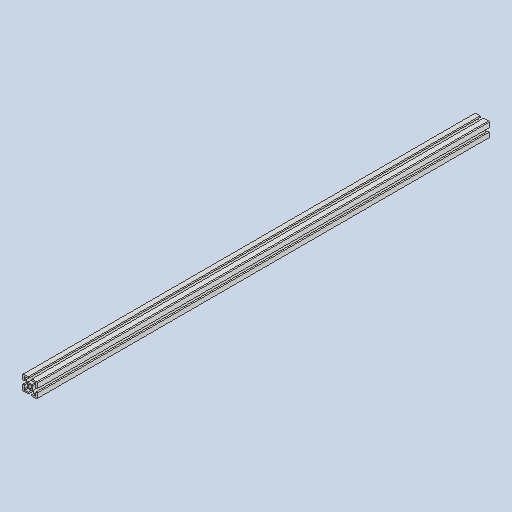
# Autodesk Inventor part: Perfil 20X20 T-622
Saved by Autodesk Inventor 2024.2 (Build 282272000, 272)
## iProperties
Created: 2024-08-23
Part Number: Perfil 20X20 T-622
Material: Generic
Document SubType Name: Modeling
Designer: ja.restrepo1
Density: 1 g/cm^3
Appearance: Default
Author: ja.restrepo1
Autodesk Inventor part; units mm, degrees
ref_plane "YZ Plane" through (0, 0, 0) normal (1, 0, 0) x (0, 1, 0)
ref_plane "XZ Plane" through (0, 0, 0) normal (0, 1, 0) x (-1, 0, 0)
ref_plane "XY Plane" through (0, 0, 0) normal (0, 0, 1) x (1, 0, 0)
sketch "Sketch1" plane through (0, 0, 0) normal (0, 0, 1) x (1, 0, 0)
  line L0 (9, 10) -> (2.5, 10)
  line L1 (-10, 9) -> (-10, 2.5)
  line L2 (-9, -10) -> (-2.5, -10)
  line L3 (10, -9) -> (10, -2.5)
  circle A0 centre (0, 0) radius 2.5
  line L4 (3.6, 3.6) -> (-3.6, 3.6) construction
  line L5 (-3.6, 3.6) -> (-3.6, -3.6) construction
  line L6 (-3.6, -3.6) -> (3.6, -3.6) construction
  line L7 (3.6, -3.6) -> (3.6, 3.6) construction
  line L8 (3.6, 3.6) -> (10, 10) construction
  line L9 (3.6, -3.6) -> (10, -10) construction
  line L10 (-3.6, -3.6) -> (-10, -10) construction
  line L11 (-10, 10) -> (-3.6, 3.6) construction
  line L12 (3.65, 2.8974) -> (8, 7.2474)
  line L13 (8, 7.2474) -> (8, 2.5)
  line L14 (8, 2.5) -> (10, 2.5)
  line L15 (10, 2.5) -> (10, -2.5) construction
  line L16 (10, -2.5) -> (8, -2.5)
  line L17 (8, -2.5) -> (8, -7.2474)
  line L18 (8, -7.2474) -> (3.65, -2.8974)
  line L19 (3.65, -2.8974) -> (3.65, 2.8974)
  line L20 (10, 2.5) -> (10, 9)
  line L21 (10, -2.5) -> (10, 2.5) construction
  line L22 (-2.5, 8) -> (-2.5, 10)
  line L23 (-7.2474, 8) -> (-2.5, 8)
  line L24 (-2.8974, 3.65) -> (-7.2474, 8)
  line L25 (2.8974, 3.65) -> (-2.8974, 3.65)
  line L26 (7.2474, 8) -> (2.8974, 3.65)
  line L27 (2.5, 8) -> (7.2474, 8)
  line L28 (2.5, 10) -> (2.5, 8)
  line L29 (-8, -2.5) -> (-10, -2.5)
  line L30 (-8, -7.2474) -> (-8, -2.5)
  line L31 (-3.65, -2.8974) -> (-8, -7.2474)
  line L32 (-3.65, 2.8974) -> (-3.65, -2.8974)
  line L33 (-8, 7.2474) -> (-3.65, 2.8974)
  line L34 (-8, 2.5) -> (-8, 7.2474)
  line L35 (-10, 2.5) -> (-8, 2.5)
  line L36 (2.5, -8) -> (2.5, -10)
  line L37 (7.2474, -8) -> (2.5, -8)
  line L38 (2.8974, -3.65) -> (7.2474, -8)
  line L39 (-2.8974, -3.65) -> (2.8974, -3.65)
  line L40 (-7.2474, -8) -> (-2.8974, -3.65)
  line L41 (-2.5, -8) -> (-7.2474, -8)
  line L42 (-2.5, -10) -> (-2.5, -8)
  line L43 (-2.5, -10) -> (2.5, -10) construction
  line L44 (2.5, -10) -> (9, -10)
  line L45 (-10, 2.5) -> (-10, -2.5) construction
  line L46 (-10, -2.5) -> (-10, -9)
  line L47 (-2.5, 10) -> (-9, 10)
  line L48 (2.5, 10) -> (-2.5, 10) construction
  arc A1 (-9, 10) -> (-10, 9) centre (-9, 9) ccw
  arc A2 (10, 9) -> (9, 10) centre (9, 9) ccw
  arc A3 (9, -10) -> (10, -9) centre (9, -9) ccw
  arc A4 (-10, -9) -> (-9, -10) centre (-9, -9) ccw
  point P0 (0, 0)
  point P1 (0, 3.6)
  point P2 (3.6, 0)
  point P3 (10, 0)
  point P4 (3.65, 0)
  point P5 (10, 0)
  point P6 (0, 3.65)
  point P7 (0, 3.65)
  point P8 (-3.65, 0)
  point P9 (0, -3.65)
  point P10 (0, 10)
  dimension "d2" = 5
  dimension "d3" = 7.2
  dimension "d4" = 7.2
  dimension "d5" = 2
  dimension "d6" = 6.35
  dimension "d7" = 4.7474
  dimension "d8" = 5
  dimension "d9" = 10
  dimension "d10" = 360
  dimension "d11" = 10
  dimension "d12" = 1
  constraints: 98 end point, 21 parallel, 16 perpendicular, 15 point on line, 8 point on circle, 8 tangent, 7 coincident, 7 midpoint, 5 centre point, 4 collinear, 4 horizontal, 4 horizontal alignment, 3 equal radius, 3 vertical alignment, 1 vertical, 65 other
  measures "d2" diameter of A0
  measures "d3" distance of L6.end L10.start
  measures "d4" distance of L10.start L5.start
  measures "d5" distance of L13.end L15.start
  measures "d6" distance between parallel lines of L15 L19
  measures "d7" distance of L16.end L17.end
  measures "d8" distance of L15.start L3.end
  measures "d9" distance from line of point (0, 0) L0
  measures "d11" distance from line of L47 point (0, 0)
  measures "d12" radius of A1
extrude "Perfil 20X20-620" add sketch "Sketch1" along normal mid plane 610
thread "M6-1" size "M6x1" class "6H" standard "ANSI Metric M Profile" length 25
thread "M6-2" size "M6x1" class "6H" standard "ANSI Metric M Profile" length 25
sketch "Sketch2" plane through (-2.8974, 10, 305) normal (0, 1, 0) x (1, 0, 0)
  line L0 (2.8974, 10) -> (2.8974, 600) construction
  point P0 (2.8974, 305)
  point P1 (2.8974, 305)
  dimension "d23" = 590
  constraints: 4 coincident, 2 end point, 1 midpoint, 1 vertical
  measures "d23" distance of L0.start L0.end
hole "BCA M5" [suppressed]
sketch "Sketch3" plane through (-2.8974, 3.65, 305) normal (0, 1, 0) x (1, 0, 0)
  line L0 (2.8974, 10) -> (2.8974, 600) construction
  point P0 (2.8974, 305)
  point P1 (2.8974, 305)
  dimension "d31" = 590
  constraints: 2 coincident, 2 end point, 1 midpoint, 1 vertical
  measures "d31" distance of L0.start L0.end
hole "M5" [suppressed]
sketch "Sketch4" plane through (-2.8974, 3.65, 305) normal (0, 1, 0) x (1, 0, 0)
  line L0 (2.8974, 10) -> (2.8974, 600) construction
  point P0 (2.8974, 305)
  point P1 (2.8974, 305)
  dimension "d39" = 590
  constraints: 2 coincident, 2 end point, 1 midpoint, 1 vertical
  measures "d39" distance of L0.start L0.end
hole "Ø5" at (0, 3.65, 295) at (0, 3.65, -295) direction (0, -1, 0) diameter 5 end through all
thread "Thread3" size "M6x1" class "6H" standard "ANSI Metric M Profile" length 15
body "Solid1"
